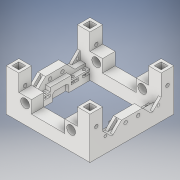
# Autodesk Inventor part: 000.101 - Частья центральная ходовой части
Saved by Autodesk Inventor 2019 (Build 230136000, 136)
## iProperties
Created: 2020-06-05
Part Number: 000.101 - Частья центральная ходовой части
Material: Пластик АБС
Document SubType Name: Modeling
Designer: Петров Иван
Density: 1.06 g/cm^3
Appearance: Белый
Author: Петров Иван
Autodesk Inventor part; units mm, degrees
ref_plane "YZ Plane" through (0, 0, 0) normal (1, 0, 0) x (0, 1, 0)
ref_plane "XZ Plane" through (0, 0, 0) normal (0, 1, 0) x (-1, 0, 0)
ref_plane "XY Plane" through (0, 0, 0) normal (0, 0, 1) x (1, 0, 0)
sketch "Эскиз1" plane through (0, 0, 0) normal (0, 1, 0) x (-1, 0, 0)
  line L0 (-50, 50) -> (0, 50)
  line L1 (0, 50) -> (0, -50)
  line L2 (0, -50) -> (-50, -50)
  line L3 (-50, -50) -> (-50, 50)
  point P0 (0, 0)
  point P1 (0, 0)
  dimension "d2" = 100
  dimension "d8" = 50
  dimension "d9" = 50
  constraints: 8 end point, 2 parallel, 1 coincident, 1 horizontal, 1 perpendicular
  measures "d2" distance of L0.end L1.end
  measures "d8" distance of L1.end L2.end
  measures "d9" distance from line of point (0, 0) L2
extrude "Выдавливание1" add sketch "Эскиз1" along normal blind 50
sketch "Эскиз2" plane through (0, 50, 0) normal (0, 1, 0) x (1, 0, 0)
  line L0 (0, 50) -> (0, -50) projected
  line L1 (0, 35) -> (35, 35)
  line L2 (35, 35) -> (35, -35)
  line L3 (35, -35) -> (0, -35)
  line L4 (0, -35) -> (0, 35)
  line L5 (50, 50) -> (0, 50) projected
  line L6 (0, -50) -> (50, -50) projected
  line L7 (50, -50) -> (50, 50) projected
  point P0 (0, 0)
  dimension "d5" = 15
  dimension "d6" = 15
  dimension "d7" = 15
  constraints: 8 end point, 2 parallel, 1 horizontal, 1 perpendicular, 1 point on line
  measures "d5" distance between parallel lines of L1 L5
  measures "d6" distance between parallel lines of L6 L3
  measures "d7" distance between parallel lines of L7 L2
extrude "Выдавливание2" cut sketch "Эскиз2" against normal through all contours L1 L2 L3 L0
sketch "Эскиз3" plane through (0, 50, 0) normal (0, 1, 0) x (1, 0, 0)
  line L0 (35, 35) -> (0, 35) projected
  line L1 (50, 50) -> (50, -50) projected
  line L2 (35, 35) -> (50, 35)
  line L3 (50, 35) -> (50, -35)
  line L4 (50, -35) -> (35, -35)
  line L5 (35, -35) -> (35, 35)
  line L6 (35, 12.5) -> (50, 12.5)
  line L7 (50, 12.5) -> (50, -12.5)
  line L8 (50, -12.5) -> (35, -12.5)
  line L9 (35, -12.5) -> (35, 12.5)
  line L10 (35, 12.5) -> (50, -12.5) construction
  line L11 (50, 12.5) -> (35, -12.5) construction
  point P0 (0, 0)
  point P1 (42.5, 0)
  dimension "d12" = 25
  constraints: 20 end point, 4 parallel, 2 horizontal, 2 midpoint, 2 perpendicular, 2 point on line, 1 coincident
  measures "d12" distance of L6.end L7.end
extrude "Выдавливание3" cut sketch "Эскиз3" against normal blind 35 contours L1 L6 L5 L2 | L1 L4 L5 L8
sketch "Эскиз4" plane through (0, 50, 0) normal (0, 1, 0) x (1, 0, 0)
  line L0 (35, -12.5) -> (50, -12.5) projected
  line L1 (50, -12.5) -> (50, 12.5) projected
  line L2 (50, 12.5) -> (35, 12.5) projected
  line L3 (35, 12.5) -> (35, -12.5) projected
  point P0 (0, 0)
extrude "Выдавливание4" cut sketch "Эскиз4" against normal blind 25
sketch "Эскиз5" plane through (0, 50, 0) normal (0, 1, 0) x (1, 0, 0)
  line L0 (35, -35) -> (35, -12.5) projected
  line L1 (35, -35) -> (0, -35)
  line L2 (0, -35) -> (0, -50)
  line L3 (0, -50) -> (35, -50)
  line L4 (35, -50) -> (35, -35)
  line L5 (35, 35) -> (0, 35) projected
  line L6 (50, 50) -> (0, 50) projected
  line L7 (0, 35) -> (35, 35)
  line L8 (35, 35) -> (35, 50)
  line L9 (35, 50) -> (0, 50)
  line L10 (0, 50) -> (0, 35)
  line L11 (35, 50) -> (20, 50)
  line L12 (20, 50) -> (20, 35)
  line L13 (20, 35) -> (35, 35)
  line L14 (35, 35) -> (35, 50)
  line L15 (0, -50) -> (50, -50) projected
  line L16 (35, -35) -> (20, -35)
  line L17 (20, -35) -> (20, -50)
  line L18 (20, -50) -> (35, -50)
  line L19 (35, -50) -> (35, -35)
  point P0 (0, 0)
  dimension "d17" = 15
  constraints: 32 end point, 8 parallel, 5 point on line, 4 horizontal, 4 perpendicular
  measures "d17" distance of L13.end L12.end
extrude "Выдавливание5" cut sketch "Эскиз5" against normal up to surface (35 mm away) contours L17 L3 L2 L1 | L5 L10 L6 L12
sketch "Эскиз6" plane through (0, 50, 0) normal (0, 1, 0) x (1, 0, 0)
  line L0 (35, -35) -> (35, -12.5)
  line L1 (35, -35) -> (0, -35)
  line L2 (0, -35) -> (0, -50)
  line L3 (0, -50) -> (35, -50)
  line L4 (35, -50) -> (35, -35)
  line L5 (35, 35) -> (0, 35)
  line L6 (50, 50) -> (0, 50)
  line L7 (0, 35) -> (35, 35)
  line L8 (35, 35) -> (35, 50)
  line L9 (35, 50) -> (0, 50)
  line L10 (0, 50) -> (0, 35)
  line L11 (35, 50) -> (20, 50)
  line L12 (20, 50) -> (20, 35)
  line L13 (20, 35) -> (35, 35)
  line L14 (35, 35) -> (35, 50)
  line L15 (0, -50) -> (50, -50)
  line L16 (35, -35) -> (20, -35)
  line L17 (20, -35) -> (20, -50)
  line L18 (20, -50) -> (35, -50)
  line L19 (35, -50) -> (35, -35)
  point P0 (0, 0)
  point P1 (0, 0)
  dimension "d20" = 15
  constraints: 40 end point, 8 parallel, 5 point on line, 4 horizontal, 4 perpendicular
  measures "d20" distance of L13.end L12.end
extrude "Выдавливание6" cut sketch "Эскиз6" against normal blind 20 contours L4 L3 L17 L1 | L5 L12 L6 L8
sketch "Эскиз7" plane through (0, 0, 50) normal (0, 0, 1) x (1, 0, 0)
  line L0 (20, 30) -> (35, 30) projected
  line L1 (20, 15) -> (20, 30) projected
  circle A0 centre (27.5, 22.5) radius 5.25
  point P0 (0, 0)
  point P1 (27.5, 30)
  point P2 (20, 22.5)
  dimension "d23" = 10.5
  dimension "d26" = 7.5
  dimension "d27" = 7.5
  constraints: 2 midpoint, 1 centre point, 1 coincident
  measures "d23" diameter of A0
  measures "d26" distance of point (27.5, 30) A0.centre
  measures "d27" distance of point (20, 22.5) A0.centre
extrude "Выдавливание7" cut sketch "Эскиз7" against normal blind 115.5
sketch "Эскиз8" plane through (50, 0, 50) normal (1, 0, 0) x (0, 0, -1)
  line L0 (37.5, 15) -> (37.5, 25) projected
  line L1 (37.5, 20) -> (62.5, 20)
  line L2 (62.5, 15) -> (62.5, 25) projected
  circle A0 centre (42.5, 20) radius 2.1
  circle A1 centre (57.5, 20) radius 2.1
  point P0 (50, 0)
  dimension "d28" = 4.2
  dimension "d29" = 4.2
  dimension "d30" = 5
  dimension "d31" = 5
  constraints: 2 centre point, 2 end point, 2 midpoint, 2 point on line
  measures "d28" diameter of A0
  measures "d29" diameter of A1
  measures "d30" distance from line of L2 A1.centre
  measures "d31" distance from line of L0 A0.centre
extrude "Выдавливание8" cut sketch "Эскиз8" against normal blind 115.5
sketch "Эскиз9" plane through (0, 25, 0) normal (0, 1, 0) x (1, 0, 0)
  line L0 (50, 12.5) -> (35, 12.5) projected
  line L1 (35, -12.5) -> (50, -12.5) projected
  line L2 (35, 12.5) -> (40.5, 12.5)
  line L3 (40.5, 12.5) -> (40.5, -12.5)
  line L4 (40.5, -12.5) -> (35, -12.5)
  line L5 (35, -12.5) -> (35, 12.5)
  point P0 (0, 0)
  dimension "d34" = 5.5
  constraints: 8 end point, 2 parallel, 1 horizontal, 1 perpendicular, 1 point on line
  measures "d34" distance of L3.end L4.end
extrude "Выдавливание9" cut sketch "Эскиз9" against normal up to surface (10 mm away)
chamfer "Фаска1" distance 10 angle 45 2 edges at (45.25, 15, 12.5) (45.25, 15, -12.5)
sketch "Эскиз10" plane through (0, 25, 0) normal (0, 1, 0) x (1, 0, 0)
  line L0 (40.5, 12.5) -> (50, 12.5) projected
  line L1 (45.25, 12.5) -> (45.25, 22.5)
  line L2 (50, 22.5) -> (40.5, 22.5) projected
  line L3 (45.25, 22.5) -> (43.74, 22.5)
  line L4 (45.25, 12.5) -> (46.76, 12.5)
  line L5 (43.74, 22.5) -> (46.76, 22.5)
  line L6 (46.76, 22.5) -> (46.76, 12.5)
  line L7 (46.76, 12.5) -> (43.74, 12.5)
  line L8 (43.74, 12.5) -> (43.74, 22.5)
  point P0 (0, 0)
  dimension "d40" = 1.51
  dimension "d41" = 1.51
  constraints: 14 end point, 2 midpoint, 2 parallel, 2 point on line, 1 horizontal, 1 perpendicular
  measures "d40" distance of L1.end L3.end
  measures "d41" distance of L4.end L1.start
extrude "Выдавливание10" cut sketch "Эскиз10" against normal up to surface (10 mm away)
ref_plane "РабПлоскость1" through (50, 25, 0) normal (0, 0, 1) x (1, 0, 0)
mirror "Зеркальное отражение1" about plane through (50, 25, 0) normal (0, 0, 1) of "Выдавливание10"
sketch "Эскиз11" plane through (0, 15, 0) normal (0, 1, 0) x (1, 0, 0)
  line L0 (40.5, 12.5) -> (43.74, 12.5) projected
  line L1 (43.74, -12.5) -> (40.5, -12.5) projected
  line L2 (40.5, -12.5) -> (35, -12.5)
  line L3 (35, -12.5) -> (35, -35)
  line L4 (35, -35) -> (40.5, -35)
  line L5 (40.5, -35) -> (40.5, -12.5)
  line L6 (35, -35) -> (35, 35) projected
  line L7 (40.5, 12.5) -> (35, 12.5)
  line L8 (35, 12.5) -> (35, 35)
  line L9 (35, 35) -> (40.5, 35)
  line L10 (40.5, 35) -> (40.5, 12.5)
  point P0 (0, 0)
  constraints: 16 end point, 4 parallel, 2 horizontal, 2 perpendicular
extrude "Выдавливание11" cut sketch "Эскиз11" against normal blind 3.3
sketch "Эскиз12" plane through (35, 0, -35) normal (-1, 0, 0) x (0, 0, 1)
  line L0 (0, 0) -> (0, 15) projected
  line L1 (70, 15) -> (70, 0) projected
  line L2 (0, 9.7) -> (70, 9.7)
  line L3 (70, 9.7) -> (70, 6.7)
  line L4 (70, 6.7) -> (0, 6.7)
  line L5 (0, 6.7) -> (0, 9.7)
  line L6 (22.5, 11.7) -> (0, 11.7) projected
  line L7 (22.5, 9.7) -> (47.5, 9.7)
  line L8 (47.5, 9.7) -> (47.5, 6.7)
  line L9 (47.5, 6.7) -> (22.5, 6.7)
  line L10 (22.5, 6.7) -> (22.5, 9.7)
  line L11 (8.75, 6.7) -> (13.75, 6.7)
  line L12 (13.75, 6.7) -> (13.75, 9.7)
  line L13 (13.75, 9.7) -> (8.75, 9.7)
  line L14 (8.75, 9.7) -> (8.75, 6.7)
  point P0 (35, 0)
  point P1 (11.25, 8.2)
  dimension "d46" = 3
  dimension "d47" = 5
  dimension "d48" = 5
  constraints: 24 end point, 6 parallel, 5 point on line, 3 horizontal, 3 perpendicular
  measures "d46" distance between parallel lines of L2 L4
  measures "d47" distance between parallel lines of L6 L4
  measures "d48" distance of L13.end L12.end
extrude "Выдавливание12" cut sketch "Эскиз12" against normal blind 5.6 contours L0 L2 L14 L4 | L12 L2 L10 L4
mirror "Зеркальное отражение2" about plane through (50, 25, 0) normal (0, 0, 1) of "Выдавливание12"
thicken "Толщина1" operation add thickness 1.4 both sides no extend neighbours yes toward (0, 1, 0) faces at (36.8333, 15, -4.1667)
sketch "Эскиз13" plane through (0, 11.7, 0) normal (0, 1, 0) x (1, 0, 0)
  line L0 (40.6, 12.5) -> (35, 12.5) projected
  line L1 (40.6, 12.5) -> (40.6, 21.25) projected
  line L2 (35, 21.25) -> (40.6, 21.25) projected
  line L3 (35, 12.5) -> (35, 21.25) projected
  line L4 (40.6, 26.25) -> (35, 26.25) projected
  line L5 (40.6, 26.25) -> (40.6, 35) projected
  line L6 (35, 35) -> (40.6, 35) projected
  line L7 (35, 26.25) -> (35, 35) projected
  circle A0 centre (37.75, 30.625) radius 1.6
  circle A1 centre (37.75, 16.875) radius 1.6
  point P0 (0, 0)
  dimension "d53" = 3.2
  dimension "d54" = 3.2
  dimension "d55" = 2.75
  dimension "d56" = 2.75
  dimension "d57" = 4.375
  dimension "d58" = 4.375
  constraints: 2 centre point
  measures "d53" diameter of A0
  measures "d54" diameter of A1
  measures "d55" distance from line of L3 A1.centre
  measures "d56" distance from line of L7 A0.centre
  measures "d57" distance from line of L2 A1.centre
  measures "d58" distance from line of L6 A0.centre
extrude "Выдавливание13" cut sketch "Эскиз13" against normal blind 5.6 contours A0 | A1
mirror "Зеркальное отражение3" about plane through (50, 25, 0) normal (0, 0, 1) of "Выдавливание13"
sketch "Эскиз14" plane through (0, 0, 0) normal (0, -1, 0) x (1, 0, 0)
  line L0 (50, 9.6) -> (50, 5.4) projected
  line L1 (50, -5.4) -> (50, -9.6) projected
  line L2 (50, -5.4) -> (40.5, -5.4) projected
  line L3 (50, -9.6) -> (40.5, -9.6) projected
  line L4 (50, 9.6) -> (40.5, 9.6) projected
  line L5 (35, 35) -> (35, -35) projected
  line L6 (35, 9.6) -> (38.4, 9.6)
  line L7 (38.4, 9.6) -> (38.4, -9.6)
  line L8 (38.4, -9.6) -> (35, -9.6)
  line L9 (35, -9.6) -> (35, 9.6)
  point P0 (0, 0)
  dimension "d61" = 3.4
  constraints: 8 end point, 2 parallel, 1 horizontal, 1 perpendicular, 1 point on line
  measures "d61" distance of L7.end L8.end
extrude "Выдавливание14" cut sketch "Эскиз14" against normal blind 10
chamfer "Фаска2" distance 2.25 angle 45 2 edges at (36.7, 10, 9.6) (36.7, 10, -9.6)
sketch "Эскиз16" plane through (0, 50, 0) normal (0, 1, 0) x (1, 0, 0)
  line L0 (35, 35) -> (50, 35) projected
  line L1 (35, 50) -> (35, 35) projected
  line L2 (38.4, 46.6) -> (46.6, 46.6)
  line L3 (46.6, 46.6) -> (46.6, 38.4)
  line L4 (46.6, 38.4) -> (38.4, 38.4)
  line L5 (38.4, 38.4) -> (38.4, 46.6)
  line L6 (38.4, 46.6) -> (46.6, 38.4) construction
  line L7 (46.6, 46.6) -> (38.4, 38.4) construction
  point P0 (0, 0)
  point P1 (42.5, 35)
  point P2 (35, 42.5)
  point P3 (42.5, 42.5)
  dimension "d67" = 8.2
  dimension "d68" = 8.2
  dimension "d71" = 7.5
  dimension "d72" = 7.5
  constraints: 12 end point, 4 midpoint, 2 parallel, 1 horizontal, 1 perpendicular
  measures "d67" distance of L3.end L4.end
  measures "d68" distance of L2.end L3.end
  measures "d71" distance of point (42.5, 35) point (42.5, 42.5)
  measures "d72" distance of point (35, 42.5) point (42.5, 42.5)
extrude "Выдавливание15" cut sketch "Эскиз16" against normal up to surface (20 mm away)
mirror "Зеркальное отражение5" about plane through (50, 25, 0) normal (0, 0, 1) of "Выдавливание15"
sketch "Эскиз17" plane through (50, 0, 50) normal (1, 0, 0) x (0, 0, -1)
  line L0 (85, 50) -> (100, 50) projected
  line L1 (92.5, 50) -> (92.5, 33.6)
  circle A0 centre (92.5, 33.6) radius 2.1
  point P0 (50, 0)
  dimension "d73" = 16.4
  dimension "d74" = 4.2
  constraints: 2 end point, 1 centre point, 1 coincident, 1 midpoint, 1 vertical
  measures "d73" distance of L1.start L1.end
  measures "d74" diameter of A0
extrude "Выдавливание16" cut sketch "Эскиз17" against normal blind 18.5
mirror "Зеркальное отражение6" about plane through (50, 25, 0) normal (0, 0, 1) of "Выдавливание16"
sketch "Эскиз21" plane through (0, 15, 0) normal (0, 1, 0) x (1, 0, 0)
  line L0 (40.5, 35) -> (50, 35) projected
  line L1 (50, 35) -> (46.76, 35)
  line L2 (46.76, 35) -> (46.76, 25)
  line L3 (46.76, 25) -> (50, 25)
  line L4 (50, 25) -> (50, 35)
  point P0 (0, 0)
  dimension "d78" = 10
  constraints: 8 end point, 2 parallel, 1 horizontal, 1 perpendicular
  measures "d78" distance of L2.end L1.end
extrude "Выдавливание17" add sketch "Эскиз21" along normal blind 10
chamfer "Фаска3" distance 10 angle 45 1 edges at (48.38, 25, -25)
sketch "Эскиз22" plane through (50, 0, 50) normal (1, 0, 0) x (0, 0, -1)
  line L0 (85, 15) -> (85, 25) projected
  line L1 (75, 15) -> (85, 15) projected
  line L2 (85, 25) -> (75, 15) projected
  line L3 (80, 20) -> (81.7678, 18.2322)
  line L4 (75, 15) -> (85, 25) projected
  circle A0 centre (81.7678, 18.2322) radius 1.6
  point P0 (50, 0)
  dimension "d84" = 2.5
  dimension "d85" = 3.2
  constraints: 2 end point, 2 perpendicular, 1 centre point, 1 coincident, 1 midpoint
  measures "d84" distance of L3.start L3.end
  measures "d85" diameter of A0
extrude "Выдавливание18" cut sketch "Эскиз22" against normal blind 10 contours A0
mirror "Зеркальное отражение7" about plane through (50, 25, 0) normal (0, 0, 1) of "Выдавливание17", "Выдавливание18", "Фаска3"
mirror "Зеркальное отражение4" about plane through (0, 0, 0) normal (1, 0, 0) of "Выдавливание1", "Выдавливание2", "Выдавливание3", "Выдавливание4", "Выдавливание5", "Выдавливание6", "Выдавливание7", "Выдавливание8", "Выдавливание9", "Фаска1", "Выдавливание10", "Зеркальное отражение1", "Выдавливание11", "Выдавливание12", "Зеркальное отражение2", "Толщина1", "Выдавливание13", "Зеркальное отражение3", "Выдавливание14", "Фаска2", "Выдавливание16", "Выдавливание15", "Зеркальное отражение5", "Зеркальное отражение6", "Выдавливание18", "Фаска3", "Выдавливание17", "Зеркальное отражение7"
ref_plane "РабПлоскость2" through (-50, 25, 0) normal (0, 0, -1) x (-1, 0, 0)
equation "\"d6\" = d5"
equation "\"d29\" = d28"
equation "\"d30\" = d31"
equation "\"d41\" = d40"
equation "\"d53\" = d54"
equation "\"d56\" = d55"
equation "\"d58\" = d57"
equation "\"d67\" = d68"
